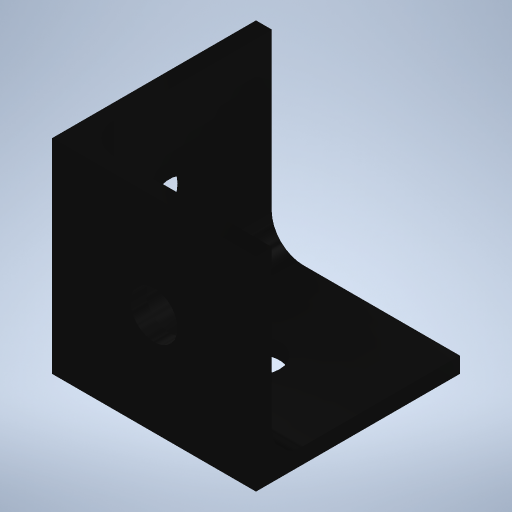
# Autodesk Inventor part: Escuadra_triple
Saved by Autodesk Inventor 2023 (Build 270158000, 158)
## iProperties
Created: 2022-12-03
Part Number: Escuadra_triple
Material: Genérico
Document SubType Name: Modeling
Designer: sergi
Density: 1 g/cm^3
Appearance: Valor por defecto
Author: sergi
Autodesk Inventor part; units mm, degrees
ref_plane "YZ Plane" through (0, 0, 0) normal (1, 0, 0) x (0, 1, 0)
ref_plane "XZ Plane" through (0, 0, 0) normal (0, 1, 0) x (-1, 0, 0)
ref_plane "XY Plane" through (0, 0, 0) normal (0, 0, 1) x (1, 0, 0)
sketch "Boceto1" plane through (0, 0, 0) normal (0, 1, 0) x (-1, 0, 0)
  line L0 (-6.5, 6.5) -> (6.5, 6.5)
  line L1 (6.5, 6.5) -> (6.5, -6.5)
  line L2 (6.5, -6.5) -> (-6.5, -6.5)
  line L3 (-6.5, -6.5) -> (-6.5, 6.5)
  line L4 (-6.5, 6.5) -> (6.5, -6.5) construction
  line L5 (6.5, 6.5) -> (-6.5, -6.5) construction
  point P0 (0, 0)
  dimension "d0" = 13
  dimension "d1" = 13
  constraints: 12 end point, 2 midpoint, 2 parallel, 1 horizontal, 1 perpendicular
  measures "d0" distance of L1.end L2.end
  measures "d1" distance of L0.end L1.end
extrude "Extrusión1" add sketch "Boceto1" along normal blind 13
shell "Vaciado1" thickness 1 removed faces 3 at (2.1667, 13, 2.1667) at (2.1667, 4.3333, -6.5) at (6.5, 4.3333, 2.1667)
fillet "Empalme1" radius 2 3 edges at (0.5, 1, 5.5) (-5.5, 1, -0.5) (-5.5, 7, 5.5)
sketch "Boceto2" plane through (-3.5, 1, 3.5) normal (0, 1, 0) x (1, 0, 0)
  line L0 (0, 10) -> (10, 10) projected
  line L1 (10, 10) -> (10, 0) projected
  point P0 (3.5, 3.5)
  point P1 (3.5, 3.5)
  dimension "d6" = 6.5
  dimension "d7" = 6.5
  measures "d6" distance from line of L0 point (3.5, 3.5)
  measures "d7" distance from line of L1 point (3.5, 3.5)
hole "Agujero1" at (0, 1, 0) direction (0, -1, 0) diameter 3 depth 3 tip angle 118
sketch "Boceto3" plane through (6.5, 13, 5.5) normal (0, 0, -1) x (-1, 0, 0)
  line L0 (0, 0) -> (10, 0) projected
  line L1 (0, -10) -> (0, 0) projected
  point P0 (6.5, -13)
  point P1 (6.5, -6.5)
  dimension "d15" = 6.5
  dimension "d16" = 6.5
  measures "d15" distance from line of L0 point (6.5, -6.5)
  measures "d16" distance from line of L1 point (6.5, -6.5)
hole "Agujero2" at (0, 6.5, 5.5) direction (0, 0, 1) diameter 3 depth 3 tip angle 118
sketch "Boceto4" plane through (-5.5, 3, -6.5) normal (1, 0, 0) x (0, 0, -1)
  line L0 (0, 10) -> (0, 0) projected
  line L1 (-10, 10) -> (0, 10) projected
  point P0 (-6.5, -3)
  point P1 (-6.5, 3.5)
  dimension "d24" = 6.5
  dimension "d25" = 6.5
  measures "d24" distance from line of L0 point (-6.5, 3.5)
  measures "d25" distance from line of L1 point (-6.5, 3.5)
hole "Agujero3" at (-5.5, 6.5, 0) direction (-1, 0, 0) diameter 3 depth 3 tip angle 118
